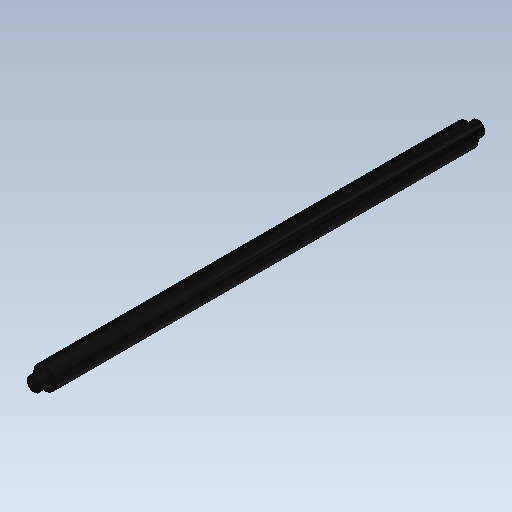
# Autodesk Inventor part: ADSK-MH-10044
Saved by Autodesk Inventor 2020.2 (Build 242310000, 310)
## iProperties
Created: 2008-03-29
Part Number: ADSK-MH-10044
Document SubType Name: Modeling
Designer: R.O'Mahony
Density: 7.86 g/cm^3
Material: Steel, Mild
Appearance: Glossy - Black
Description: Roller Shaft
Engineer: Demir Ali
Checked By: Demir Ali
Company: Autodesk Ltd
Author: R.O'Mahony
Keywords: Roller Conveyor
Revision Number: A
Autodesk Inventor part; units mm, degrees
ref_plane "YZ Plane" through (0, 0, 0) normal (1, 0, 0) x (0, 1, 0)
ref_plane "XZ Plane" through (0, 0, 0) normal (0, 1, 0) x (-1, 0, 0)
ref_plane "XY Plane" through (0, 0, 0) normal (0, 0, 1) x (1, 0, 0)
sketch "Sketch1" plane through (0, 0, 0) normal (0, 0, 1) x (1, 0, 0)
  circle A0 centre (0, 0) radius 9.5
  dimension "d0" = 19
  constraints: 1 centre point
  measures "d0" diameter of A0
extrude "Extrusion1" add sketch "Sketch1" along normal mid plane 350
sketch "Sketch2" plane through (0, 0, 175) normal (0, 0, 1) x (1, 0, 0)
  circle A0 centre (0, 0) radius 9.5 projected
  circle A1 centre (0, 0) radius 6
  dimension "d3" = 12
  constraints: 1 centre point, 1 coincident
  measures "d3" diameter of A1
extrude "Extrusion2" add sketch "Sketch2" along normal blind 9 contours A1
sketch "Sketch3" plane through (0, 0, -175) normal (0, 0, -1) x (-1, 0, 0)
  circle A0 centre (0, 0) radius 9.5 projected
  circle A1 centre (0, 0) radius 6
  dimension "d6" = 12
  constraints: 1 centre point, 1 coincident
  measures "d6" diameter of A1
extrude "Extrusion3" add sketch "Sketch3" along normal blind 9 contours A1
body "Solid1"
